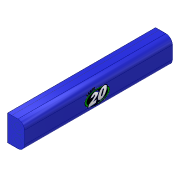
# Autodesk Inventor part: SideBumper
Saved by Autodesk Inventor 2018 (Build 220112000, 112)
## iProperties
Created: 2020-02-05
Part Number: SideBumper
Material: Wood (Birch)
Document SubType Name: Modeling
Designer: Myers
Mass: 3043.93 g
Surface Area: 12933.7 cm^2
Volume: 5534.42 cm^3
Density: 0.55 g/cm^3
Appearance: Birch - Natural Polished
Author: Myers
Autodesk Inventor part; units mm, degrees
ref_plane "YZ Plane" through (0, 0, 0) normal (1, 0, 0) x (0, 1, 0)
ref_plane "XZ Plane" through (0, 0, 0) normal (0, 1, 0) x (-1, 0, 0)
ref_plane "XY Plane" through (0, 0, 0) normal (0, 0, 1) x (1, 0, 0)
sketch "Sketch1" plane through (0, 0, 0) normal (0, 0, 1) x (1, 0, 0)
  line L0 (0, 0) -> (19.05, 0)
  line L1 (19.05, 0) -> (19.05, -127)
  line L2 (19.05, -127) -> (0, -127)
  line L3 (0, -127) -> (0, 0)
  circle A0 centre (50.8, -31.75) radius 31.75
  circle A1 centre (50.8, -31.75) radius 15.875
  circle A2 centre (50.8, -95.25) radius 15.875
  circle A3 centre (50.8, -95.25) radius 31.75
  dimension "d0" = 19.05
  dimension "d1" = 127
  dimension "d2" = 31.75
  constraints: 8 end point, 5 tangent, 4 centre point, 2 equal radius, 2 parallel, 1 coincident, 1 concentric, 1 horizontal, 1 perpendicular
  measures "d0" distance of L0.start L0.end
  measures "d1" distance of L2.end L0.start
  measures "d2" diameter of A1
extrude "Extrusion1" add sketch "Sketch1" along normal blind 736.6 contours L0 L1 L2 L3
extrude "Extrusion2" add sketch "Sketch1" along normal up to surface (736.6 mm away) separate body contours A0 | A3
sketch "Sketch2" plane through (0, 0, 0) normal (0, 0, -1) x (-1, 0, 0)
  line L0 (-19.05, -127) -> (0, -127) projected
  line L1 (0, -127) -> (0, 0) projected
  line L2 (0, 0) -> (-50.8, 0)
  circle A0 centre (-50.8, -31.75) radius 31.75 projected
  line L3 (0, 0) -> (0, -127) projected
  line L4 (0, 0) -> (0, -127)
  line L5 (0, -127) -> (-50.8, -127)
  circle A1 centre (-50.8, -95.25) radius 31.75 projected
  arc A2 (-82.55, -95.25) -> (-50.8, -127) centre (-50.8, -95.25) ccw
  arc A3 (-50.8, 0) -> (-82.55, -31.75) centre (-50.8, -31.75) ccw
  line L6 (-82.55, -31.75) -> (-82.55, -95.25)
  arc A4 (-83.3628, -95.25) -> (-50.8, -127.8128) centre (-50.8, -95.25) ccw
  line L7 (-50.8, -127.8128) -> (0.8128, -127.8128)
  line L8 (0.8128, -127.8128) -> (0.8128, 0.8128)
  line L9 (0.8128, 0.8128) -> (-50.8, 0.8128)
  arc A5 (-50.8, 0.8128) -> (-83.3628, -31.75) centre (-50.8, -31.75) ccw
  line L10 (-83.3628, -31.75) -> (-83.3628, -95.25)
  point P0 (-50.8, -63.5)
  dimension "d7" = 0.8128
  constraints: 16 end point, 10 point on circle, 4 centre point, 4 tangent, 2 concentric, 1 perpendicular, 5 other
  measures "d7" distance between parallel lines of L10 L6
extrude "Extrusion3" add sketch "Sketch2" against normal up to surface (736.6 mm away) separate body
sketch "Sketch3" plane through (0, 0, 0) normal (0, 0, -1) x (-1, 0, 0)
  arc A0 (-83.3628, -95.25) -> (-50.8, -127.8128) centre (-50.8, -95.25) ccw projected
  line L0 (-50.8, -127.8128) -> (0.8128, -127.8128) projected
  line L1 (0.8128, -127.8128) -> (0.8128, 0.8128) projected
  line L2 (0.8128, 0.8128) -> (-50.8, 0.8128) projected
  arc A1 (-50.8, 0.8128) -> (-83.3628, -31.75) centre (-50.8, -31.75) ccw projected
  line L3 (-83.3628, -31.75) -> (-83.3628, -95.25) projected
extrude "Extrusion4" add sketch "Sketch3" along normal blind 0.8128 bodies 3
sketch "Sketch5" plane through (-0.8128, -127.8128, 736.6) normal (0, 0, 1) x (1, 0, 0)
  line L0 (51.6128, 0) -> (0, 0) projected
  arc A0 (51.6128, 0) -> (84.1756, 32.5628) centre (51.6128, 32.5628) ccw projected
  line L1 (84.1756, 96.0628) -> (84.1756, 32.5628) projected
  arc A1 (84.1756, 96.0628) -> (51.6128, 128.6256) centre (51.6128, 96.0628) ccw projected
  line L2 (0, 128.6256) -> (51.6128, 128.6256) projected
  line L3 (0, 0) -> (0, 128.6256) projected
extrude "Extrusion5" add sketch "Sketch5" along normal blind 0.8128 bodies 3
sketch "Sketch6" plane through (83.3628, -95.25, -0.8128) normal (1, 0, 0) x (0, 0, -1)
  line L0 (-438.2681, 74.6205) -> (-311.8686, 74.6205) construction
  line L1 (-311.8686, 74.6205) -> (-311.8686, -8.8099) construction
  line L2 (-311.8686, -8.8099) -> (-438.2681, -8.8099) construction
  line L3 (-438.2681, -8.8099) -> (-438.2681, 74.6205) construction
  point P0 (-0.8128, 95.25)
  constraints: 2 other
decal "Decal1"
body "Solid1"
body "Solid2"
body "Solid3"
